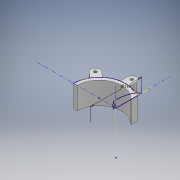
# Autodesk Inventor part: Gehäuse
Saved by Autodesk Inventor 2017 (Build 210142000, 142)
## iProperties
Created: 2019-05-27
Part Number: Gehäuse
Material: Generic
Document SubType Name: Modeling
Designer: Ole Simmering
Density: 1 g/cm^3
Appearance: Default
Author: Ole Simmering
Autodesk Inventor part; units mm, degrees
ref_plane "YZ Plane" through (0, 0, 0) normal (1, 0, 0) x (0, 1, 0)
ref_plane "XZ Plane" through (0, 0, 0) normal (0, 1, 0) x (-1, 0, 0)
ref_plane "XY Plane" through (0, 0, 0) normal (0, 0, 1) x (1, 0, 0)
sketch "Sketch1" plane through (0, 0, 0) normal (0, 0, 1) x (1, 0, 0)
  line L0 (-110.5, 0) -> (110.5, 0) construction
  line L1 (0, 110.5) -> (0, -110.5) construction
  line L2 (-110.5, 110.5) -> (110.5, 110.5) construction
  line L3 (110.5, 110.5) -> (110.5, -110.5) construction
  line L4 (110.5, -110.5) -> (-110.5, -110.5) construction
  line L5 (-110.5, -110.5) -> (-110.5, 110.5) construction
  circle A0 centre (-37.5, 0) radius 37.5 construction
  circle A1 centre (37.5, 0) radius 37.5 construction
  arc A2 (-2.1447, 35.3553) -> (-87.5, 0) centre (-37.5, 0) ccw
  arc A3 (-2.1447, 35.3553) -> (0, 34.467) centre (0, 37.5) ccw
  line L6 (-37.5, 0) -> (-2.1447, 35.3553) construction
  arc A4 (-47.5716, 57.1188) -> (-74.8373, 44.3838) centre (-37.5, 0) ccw
  arc A5 (-12.404, 52.2895) -> (-27.5, 57.1314) centre (-37.5, 0) ccw
  arc A6 (-12.404, 52.2895) -> (0, 49.467) centre (0, 78.1341) ccw
  line L7 (-37.5, 0) -> (-110.5, 61.2543) construction
  line L8 (-37.5, 0) -> (20.5, 0) construction
  line L9 (-37.5, 0) -> (-37.5, 110.5) construction
  line L10 (-87.6931, 29.0629) -> (-99.8491, 39.2631)
  arc A7 (-86.9934, 54.5839) -> (-99.8491, 39.2631) centre (-93.4212, 46.9235) ccw
  line L11 (-86.9934, 54.5839) -> (-74.8373, 44.3838)
  circle A8 centre (-93.4212, 46.9235) radius 3.3
  line L12 (-97.844, 50.6346) -> (-92.4187, 52.6093) construction
  line L13 (-92.4187, 52.6093) -> (-87.9959, 48.8981) construction
  line L14 (-87.9959, 48.8981) -> (-88.9985, 43.2124) construction
  line L15 (-88.9985, 43.2124) -> (-94.4238, 41.2377) construction
  line L16 (-94.4238, 41.2377) -> (-98.8466, 44.9488) construction
  line L17 (-98.8466, 44.9488) -> (-97.844, 50.6346) construction
  line L18 (-47.5, 57.1314) -> (-47.5, 73)
  line L19 (-27.5, 73) -> (-27.5, 57.1314)
  line L20 (-32.5, 70.1132) -> (-37.5, 67.2265) construction
  line L21 (-37.5, 78.7735) -> (-32.5, 75.8868) construction
  line L22 (-37.5, 67.2265) -> (-42.5, 70.1132) construction
  line L23 (-42.5, 75.8868) -> (-37.5, 78.7735) construction
  arc A9 (-27.5, 73) -> (-47.5, 73) centre (-37.5, 73) ccw
  line L24 (-32.5, 75.8868) -> (-32.5, 70.1132) construction
  circle A10 centre (-37.5, 73) radius 3.3
  line L25 (-42.5, 70.1132) -> (-42.5, 75.8868) construction
  line L26 (-37.5, 0) -> (-2.1447, -35.3553) construction
  line L27 (0, 49.467) -> (0, 34.467)
  arc A11 (-27.5, 57.1314) -> (-47.5, 57.1314) centre (-37.5, 0) ccw construction
  arc A12 (-47.5, 57.1314) -> (-47.5716, 57.1188) centre (-37.5, 0) ccw
  arc A13 (-74.8373, 44.3838) -> (-87.6931, 29.0629) centre (-37.5, 0) ccw construction
  arc A14 (-87.6931, 29.0629) -> (-95.5, 0) centre (-37.5, 0) ccw
  line L28 (-95.5, 0) -> (-87.5, 0)
  point P0 (0, 0)
  point P1 (0, 0)
  point P2 (0, 0)
  point P3 (-81.9306, 37.2817)
  point P4 (-37.5, 58)
  dimension "d10" = 75
  dimension "d7" = 221
  dimension "d8" = 221
  dimension "d9" = 75
  dimension "d11" = 50
  dimension "d12" = 135
  dimension "d13" = 8
  dimension "d14" = 15
  dimension "d15" = 140
  dimension "d17" = 10
  dimension "d19" = 6.6
  dimension "d20" = 15
  dimension "d21" = 10
  dimension "d24" = 50
  constraints: 58 end point, 26 point on circle, 14 centre point, 10 point on line, 9 coincident, 7 midpoint, 4 parallel, 4 tangent, 3 horizontal, 2 collinear, 2 line through centre, 2 vertical, 1 horizontal alignment, 1 perpendicular, 1 symmetric about line, 44 other
  measures "d7" distance between parallel lines of L4 L2
  measures "d8" distance between parallel lines of L3 L5
  measures "d9" diameter of A0
  measures "d11" radius of A2
  measures "d12" angle of L6 L0
  measures "d13" radial gap between concentric circles of A4 A2
  measures "d14" distance of L27.end L27.start
  measures "d15" angle of L8 L7
  measures "d17" radius of A7
  measures "d19" diameter of A8
  measures "d20" distance of A7.centre point (-81.931, 37.282)
  measures "d21" distance between parallel lines of L16 L13
extrude "Extrusion1" add sketch "Sketch1" along normal blind 50
sketch "Sketch4" plane through (0, 0, 50) normal (0, 0, 1) x (1, 0, 0)
  line L0 (0, 0) -> (0, 122) construction
  line L1 (0, 0) -> (-181, 0) construction
  arc A0 (-87.6931, 29.0629) -> (-95.5, 0) centre (-37.5, 0) ccw construction
  arc A1 (-12.404, 52.2895) -> (-95.5, 0) centre (-37.5, 0) ccw
  arc A2 (-12.404, 52.2895) -> (0, 49.467) centre (0, 78.1341) ccw projected
  line L2 (0, 49.467) -> (0, 0)
  arc A3 (-87.6931, 29.0629) -> (-95.5, 0) centre (-37.5, 0) ccw projected
  constraints: 6 end point, 2 coincident, 2 point on circle, 2 vertical, 1 centre point, 1 horizontal, 1 point on line
sketch "Sketch5" plane through (0, 34.467, 0) normal (1, 0, 0) x (0, 0, -1)
  arc A0 (-50, 23.533) -> (-66, -34.467) centre (47.125, -34.467) ccw
  line L0 (-50, -34.467) -> (-50, 15.533) construction
  line L1 (-50, -34.467) -> (-94, -34.467) construction
  line L2 (0, -34.467) -> (-50, -34.467) construction
  line L3 (-50, 22.6644) -> (-50, 38.533) projected
  dimension "d28" = 116
  dimension "d29" = 16
  constraints: 2 end point, 2 point on circle, 2 point on line, 1 centre point, 1 collinear, 1 horizontal, 1 line through centre
  measures "d28" diameter of A0.start L1
  measures "d29" distance of L0.start A0.end
equation "\"d10\" = d9"
body "Solid1"
